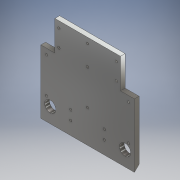
# Autodesk Inventor part: Podstawa_All_in_One_5mm
Saved by Autodesk Inventor 2017 (Build 210142000, 142)
## iProperties
Created: 2016-11-09
Part Number: Podstawa_All_in_One_5mm
Material: Generic
Document SubType Name: Modeling
Designer: Shichi
Density: 1 g/cm^3
Appearance: Chrome - Polished
Author: Shichi
Autodesk Inventor part; units mm, degrees
ref_plane "YZ Plane" through (0, 0, 0) normal (1, 0, 0) x (0, 1, 0)
ref_plane "XZ Plane" through (0, 0, 0) normal (0, 1, 0) x (-1, 0, 0)
ref_plane "XY Plane" through (0, 0, 0) normal (0, 0, 1) x (1, 0, 0)
sketch "Sketch1" plane through (0, 0, 0) normal (0, 1, 0) x (-1, 0, 0)
  line L0 (35, 35) -> (35, 3)
  line L1 (9, 3) -> (35, 3) construction
  line L2 (0, 3) -> (9, 3) construction
  line L3 (35, 3) -> (50, 3)
  line L4 (0, -35) -> (0, 35)
  line L5 (0, -35) -> (50, -35)
  line L6 (0, 35) -> (35, 35)
  line L7 (50, -35) -> (50, 3)
  line L8 (30.7, 28.05) -> (35, 28.05) construction
  line L9 (30.7, 28.05) -> (30.7, 9.95) construction
  line L10 (30.7, 9.95) -> (30.7, 3) construction
  circle A0 centre (30.7, 9.95) radius 1.25
  circle A1 centre (30.7, 28.05) radius 1.25
  circle A2 centre (44, -3) radius 1.25
  arc A3 (0, -31.25) -> (0, -28.75) centre (0, -30) ccw
  arc A4 (0, 6.45) -> (0, 8.95) centre (0, 7.7) ccw
  arc A5 (0, 28.05) -> (0, 30.55) centre (0, 29.3) ccw
  line L11 (0, 29.3) -> (30.7, 29.3) construction
  line L12 (50, -35) -> (50, -65)
  line L13 (50, -65) -> (0, -65)
  line L14 (0, -35) -> (0, -65)
  circle A6 centre (44, -41) radius 1.25
  circle A7 centre (18, -41) radius 1.25
  circle A8 centre (18, -51) radius 1.25
  point P0 (0, 0)
  point P1 (-50, 0)
  point P2 (0, 0)
  dimension "d26" = 2.5
  dimension "d6" = 32
  dimension "d9" = 26
  dimension "d10" = 9
  dimension "d11" = 50
  dimension "d12" = 70
  dimension "d14" = 4.3
  dimension "d15" = 18.1
  dimension "d20" = 6.95
  dimension "d25" = 2.5
  dimension "d32" = 2.5
  dimension "d33" = 2.5
  dimension "d35" = 2.5
  dimension "d36" = 30
  dimension "d37" = 6
  dimension "d38" = 6
  dimension "d39" = 32
  dimension "d40" = 10
  dimension "d41" = 2.5
  dimension "d42" = 2.5
  dimension "d43" = 2.5
  dimension "d55" = 6
  dimension "d56" = 6
  dimension "d57" = 2.5
  dimension "d58" = 5
  dimension "d59" = 2.25
  constraints: 28 end point, 9 vertical alignment, 8 centre point, 6 horizontal alignment, 6 point on circle, 4 coincident, 4 horizontal, 4 vertical, 2 perpendicular, 2 point on line, 1 parallel, 14 other
  measures "d6" distance of L0.start L0.end
  measures "d9" distance of L1.start L0.end
  measures "d10" distance of L2.start L1.start
  measures "d11" distance of L5.start L5.end
  measures "d12" distance of L5.start L6.start
  measures "d14" distance of L8.start L8.end
  measures "d15" distance of L8.start L9.end
  measures "d20" distance of L10.start L10.end
  measures "d25" diameter of A0
  measures "d32" diameter of A3
  measures "d33" diameter of A4
  measures "d35" diameter of A5
  measures "d36" distance of L5.end L12.end
  measures "d37" distance from line of L12 A6.centre
  measures "d38" distance from line of L5 A6.centre
  measures "d39" distance from line of L12 A7.centre
  measures "d40" distance of A7.centre A8.centre
  measures "d41" diameter of A8
  measures "d42" diameter of A7
  measures "d43" diameter of A6
  measures "d55" distance from line of L7 A2.centre
  measures "d56" distance from line of L3 A2.centre
  measures "d57" diameter of A2
  measures "d58" distance from line of L5 A3.centre
  measures "d59" vertical distance of A4.centre L9.end
extrude "Extrusion1" add sketch "Sketch1" along normal blind 5 contours L0 L3 L7 L5 L4 A3 A4 A5 L6 | A5 L4 | L12 L13 L14 L5 | A4 L4 | L4 A3 | A0 | A1 | A2
extrude "Extrusion4" cut sketch "Sketch1" along normal through all contours A5 L4 | A4 L4 | L4 A3 | A0 | A1 | A2
mirror "Mirror1" about plane through (0, 0, 0) normal (1, 0, 0) of "Extrusion1", "Extrusion4"
sketch "Sketch4" plane through (-50, 0, -65) normal (-1, 0, 0) x (0, 0, 1)
  line L0 (0, 5) -> (68, 5) projected
  line L1 (0, 5) -> (5, 5)
  line L2 (0, 0) -> (68, 0) projected
  line L3 (5, 5) -> (0, 0)
  line L4 (0, 0) -> (0, 5) projected
  line L5 (0, 0) -> (0, 5)
  point P0 (65, 0)
  dimension "d44" = 5
  constraints: 6 end point, 1 collinear, 1 point on line
  measures "d44" distance of L0.start L1.end
extrude "Extrusion5" cut sketch "Sketch4" against normal through all
sketch "Sketch5" plane through (0, 5, 0) normal (0, 1, 0) x (1, 0, 0)
  circle A0 centre (-40, 49) radius 6
  line L0 (-50, 60) -> (-50, -3) projected
  line L1 (50, 60) -> (-50, 60) projected
  point P0 (0, 0)
  dimension "d50" = 10
  dimension "d51" = 11
  dimension "d52" = 12
  constraints: 1 centre point
  measures "d50" distance from line of L0 A0.centre
  measures "d51" distance from line of L1 A0.centre
  measures "d52" diameter of A0
extrude "Extrusion6" cut sketch "Sketch5" against normal through all
mirror "Mirror2" about plane through (0, 0, 0) normal (1, 0, 0) of "Extrusion6"
body "Solid1"
